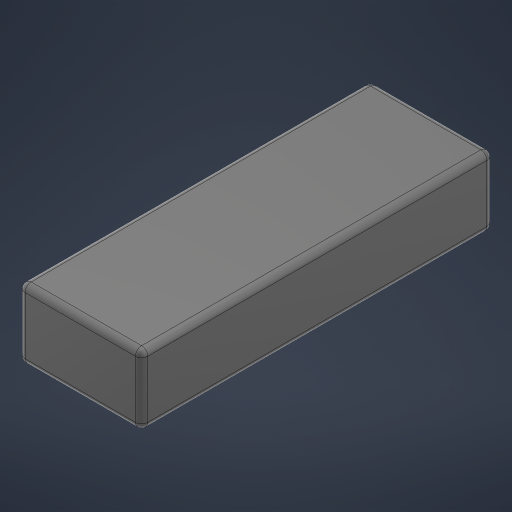
# Autodesk Inventor part: Battery_Noir3s1300mah
Saved by Autodesk Inventor 2024.2 (Build 282272000, 272)
## iProperties
Created: 2023-12-22
Part Number: Battery_Noir3s1300mah
Material: 一般
Document SubType Name: Modeling
Designer: Hanaoka
Density: 1 g/cm^3
Appearance: 既定
Author: Hanaoka
Autodesk Inventor part; units mm, degrees
ref_plane "YZ Plane" through (0, 0, 0) normal (1, 0, 0) x (0, 1, 0)
ref_plane "XZ Plane" through (0, 0, 0) normal (0, 1, 0) x (-1, 0, 0)
ref_plane "XY Plane" through (0, 0, 0) normal (0, 0, 1) x (1, 0, 0)
sketch "スケッチ1" plane through (0, 0, 0) normal (0, 1, 0) x (-1, 0, 0)
  line L0 (-15, 43) -> (15, 43)
  line L1 (15, 43) -> (15, -43)
  line L2 (15, -43) -> (-15, -43)
  line L3 (-15, -43) -> (-15, 43)
  line L4 (-15, 43) -> (15, -43) construction
  line L5 (15, 43) -> (-15, -43) construction
  point P0 (0, 0)
  dimension "d0" = 86
  dimension "d1" = 30
  constraints: 12 end point, 2 midpoint, 2 parallel, 1 horizontal, 1 perpendicular
  measures "d0" distance of L0.end L1.end
  measures "d1" distance of L1.end L2.end
extrude "押し出し1" add sketch "スケッチ1" along normal blind 17
fillet "フィレット1" radius 1.5 12 edges at (-15, 8.5, 43) (0, 17, 43) (0, 0, 43) (15, 8.5, 43) (15, 0, 0) (15, 17, 0) (0, 17, -43) (-15, 8.5, -43) (-15, 17, 0) (-15, 0, 0) (0, 0, -43) (15, 8.5, -43)
